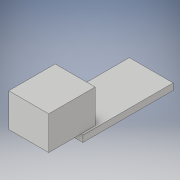
# Autodesk Inventor part: Smaller ethernet
Saved by Autodesk Inventor 2018 (Build 220112000, 112)
## iProperties
Created: 2019-09-27
Part Number: Smaller ethernet
Material: Generic
Document SubType Name: Modeling
Designer: Jacob
Density: 1 g/cm^3
Appearance: Default
Author: Jacob
Autodesk Inventor part; units mm, degrees
ref_plane "YZ Plane" through (0, 0, 0) normal (1, 0, 0) x (0, 1, 0)
ref_plane "XZ Plane" through (0, 0, 0) normal (0, 1, 0) x (-1, 0, 0)
ref_plane "XY Plane" through (0, 0, 0) normal (0, 0, 1) x (1, 0, 0)
sketch "Sketch1" plane through (0, 0, 0) normal (0, 1, 0) x (-1, 0, 0)
  line L0 (8.5, 17.5) -> (-8.5, 17.5)
  line L1 (-8.5, 17.5) -> (-8.5, -17.5)
  line L2 (-8.5, -17.5) -> (8.5, -17.5)
  line L3 (8.5, -17.5) -> (8.5, 17.5)
  line L4 (8.5, 17.5) -> (-8.5, -17.5) construction
  line L5 (-8.5, 17.5) -> (8.5, -17.5) construction
  point P0 (0, 0)
  dimension "d0" = 17
  dimension "d1" = 35
  constraints: 12 end point, 2 midpoint, 2 parallel, 1 horizontal, 1 perpendicular
  measures "d0" distance of L1.end L2.end
  measures "d1" distance of L2.end L0.start
extrude "Extrusion1" add sketch "Sketch1" along normal blind 2.5
sketch "Sketch2" plane through (0, 2.5, 0) normal (0, 1, 0) x (1, 0, 0)
  line L0 (-8.5, 17.5) -> (-8.5, -17.5) projected
  line L1 (-8.5, -12) -> (8.5, -12) construction
  line L2 (8.5, -17.5) -> (8.5, 17.5) projected
  line L3 (-8.5, -17.5) -> (8.5, -17.5) projected
  line L4 (0, 0) -> (0, -52.8122) construction
  line L5 (-7.75, -30) -> (7.75, -30)
  line L6 (7.75, -30) -> (7.75, -12)
  line L7 (7.75, -12) -> (-7.75, -12)
  line L8 (-7.75, -12) -> (-7.75, -30)
  line L9 (-7.75, -30) -> (7.75, -12) construction
  line L10 (7.75, -30) -> (-7.75, -12) construction
  point P0 (0, -21)
  dimension "d4" = 5.5
  dimension "d5" = 0
  dimension "d6" = 15.5
  dimension "d7" = 18
  constraints: 16 end point, 3 point on line, 2 horizontal, 2 midpoint, 2 parallel, 1 perpendicular, 1 vertical
  measures "d4" distance between parallel lines of L1 L3
  measures "d5" distance between parallel lines of L1 L7
  measures "d6" distance of L5.start L5.end
  measures "d7" distance of L5.end L6.end
extrude "Extrusion2" add sketch "Sketch2" along normal blind 13
body "Solid1"
